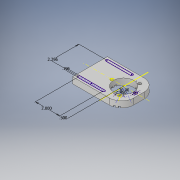
# Autodesk Inventor part: tri_mount
Saved by Autodesk Inventor 2017 (Build 210142000, 142)
## iProperties
Created: 2017-03-10
Part Number: tri_mount
Material: Generic
Document SubType Name: Modeling
Designer: richp
Density: 1 g/cm^3
Appearance: Default
mount_radius: 0.964 in
fov_diameter: 0.300 in
tri_angle: 120.00 deg
hole_diameter: 1.639 in
main_aperture_diameter: 1.639 in
Author: richp
Autodesk Inventor part; units mm, degrees
ref_plane "YZ Plane" through (0, 0, 0) normal (1, 0, 0) x (0, 1, 0)
ref_plane "XZ Plane" through (0, 0, 0) normal (0, 1, 0) x (-1, 0, 0)
ref_plane "XY Plane" through (0, 0, 0) normal (0, 0, 1) x (1, 0, 0)
sketch "Sketch1" plane through (0, 0, 0) normal (0, 1, 0) x (-1, 0, 0)
  line L0 (-54.2742, 0) -> (84.3226, 0) construction
  line L1 (-6.35, -36.068) -> (69.85, -36.068)
  line L2 (69.85, -36.068) -> (69.85, 36.068)
  line L3 (69.85, 36.068) -> (-6.35, 36.068)
  line L4 (-31.75, 10.668) -> (-31.75, -10.668)
  circle A0 centre (0, 0) radius 17 construction
  circle A1 centre (0, 0) radius 20.81
  line L5 (0, 0) -> (-18.9066, 32.7472) construction
  circle A2 centre (0, 0) radius 3.81 construction
  arc A3 (-6.35, 36.068) -> (-31.75, 10.668) centre (-6.35, 10.668) ccw
  arc A4 (-31.75, -10.668) -> (-6.35, -36.068) centre (-6.35, -10.668) ccw
  circle A5 centre (-12.2465, 21.2116) radius 1.6256
  line L6 (0, 0) -> (31.1733, 53.9938) construction
  circle A6 centre (24.493, 0) radius 1.6256
  circle A7 centre (-12.2465, -21.2116) radius 1.6256
  circle A8 centre (-12.2465, 21.2116) radius 3.175 construction
  line L7 (-57.1489, 10.668) -> (-67.0521, 10.668)
  line L8 (-67.0521, 10.668) -> (-67.0521, -7.3902)
  line L9 (-67.0521, -7.3902) -> (-57.1489, -7.3902)
  line L10 (-57.1489, -7.3902) -> (-57.1489, 10.668)
  point P0 (-31.75, -36.068)
  point P1 (-31.75, 36.068)
  dimension "d0" = 72.136
  dimension "d1" = 101.6
  dimension "d2" = 34
  dimension "d3" = 3.81
  dimension "d4" = 31.75
  dimension "tri_angle" = 120
  dimension "fov_diameter" = 7.62
  dimension "d9" = 25.4
  dimension "d12" = 3.2512
  dimension "mount_radius" = 24.493
  dimension "d14" = 60
  dimension "d25" = 6.35
  dimension "main_aperture_diameter" = 41.62
  dimension "d67" = 2.0574
  dimension "d68" = 10.94
  constraints: 22 end point, 9 centre point, 6 point on line, 5 point on circle, 4 coincident, 4 parallel, 4 tangent, 3 horizontal, 2 perpendicular, 2 symmetric about line, 1 equal radius, 3 other
  measures "d0" distance of point (-31.75, 36.068) point (-31.75, -36.068)
  measures "d1" distance of L2.end point (-31.75, 36.068)
  measures "d2" diameter of A0
  measures "d3" radial gap between concentric circles of A1 A0
  measures "d4" distance from line of L5.start L4
  measures "tri_angle" angle of L0 L5
  measures "fov_diameter" diameter of A2
  measures "d9" radius of A3
  measures "d12" diameter of A5
  measures "mount_radius" distance of L5.start A5.centre
  measures "d14" angle of L0 L6
  measures "d25" diameter of A8
  measures "main_aperture_diameter" diameter of A1
  measures "d68" distance edge to line of A1 L4
extrude "Extrusion2" add sketch "Sketch1" against normal blind 12.7 contours A4 L4 A3 L3 L2 L1
sketch "Sketch2" plane through (0, -12.7, 0) normal (0, -1, 0) x (1, 0, 0)
  line L0 (0, 0) -> (-53.7265, 0) construction
  circle A0 centre (0, 0) radius 20.81 projected
  circle A1 centre (12.2465, -21.2116) radius 1.6256 projected
  circle A2 centre (-24.493, 0) radius 1.6256 projected
  circle A3 centre (12.2465, 21.2116) radius 1.6256 projected
  line L1 (-69.85, 36.068) -> (-69.85, -36.068) projected
  line L2 (6.35, 36.068) -> (-69.85, 36.068) projected
  arc A4 (31.75, 10.668) -> (6.35, 36.068) centre (6.35, 10.668) ccw projected
  line L3 (31.75, -10.668) -> (31.75, 10.668) projected
  arc A5 (6.35, -36.068) -> (31.75, -10.668) centre (6.35, -10.668) ccw projected
  line L4 (-69.85, -36.068) -> (6.35, -36.068) projected
  line L5 (54.2742, 0) -> (-84.3226, 0) construction
  line L6 (0, 0) -> (-31.1733, 53.9938) construction
  circle A6 centre (0, 0) radius 17 construction
  circle A7 centre (0, 0) radius 3.81 construction
  line L7 (0, 0) -> (18.9066, 32.7472) construction
  line L8 (41.6502, 64.7743) -> (11.4877, 12.5313) construction
  line L9 (11.4877, 12.5313) -> (41.6502, 64.7743) construction
  line L10 (10.1129, 13.325) -> (40.2754, 65.568)
  line L11 (43.025, 63.9805) -> (12.8625, 11.7375)
  arc A8 (10.1129, 13.325) -> (12.8625, 11.7375) centre (11.4877, 12.5313) ccw
  arc A9 (43.025, 63.9805) -> (40.2754, 65.568) centre (41.6502, 64.7743) ccw
  line L12 (6.4834, 15.4205) -> (36.6459, 67.6635)
  line L13 (33.8962, 69.251) -> (3.7337, 17.008)
  arc A10 (3.7337, 17.008) -> (6.4834, 15.4205) centre (5.1086, 16.2143) ccw
  arc A11 (36.6459, 67.6635) -> (33.8962, 69.251) centre (35.2711, 68.4573) ccw
  line L14 (10.1129, -13.325) -> (40.2754, -65.568)
  line L15 (43.025, -63.9805) -> (12.8625, -11.7375)
  arc A12 (12.8625, -11.7375) -> (10.1129, -13.325) centre (11.4877, -12.5313) ccw
  arc A13 (40.2754, -65.568) -> (43.025, -63.9805) centre (41.6502, -64.7743) ccw
  arc A14 (33.8962, -69.251) -> (36.6459, -67.6635) centre (35.2711, -68.4573) ccw
  line L16 (33.8962, -69.251) -> (3.7337, -17.008)
  arc A15 (6.4834, -15.4205) -> (3.7337, -17.008) centre (5.1086, -16.2143) ccw
  line L17 (6.4834, -15.4205) -> (36.6459, -67.6635)
  line L18 (-16.5962, -2.0955) -> (-76.9212, -2.0955)
  line L19 (-76.9212, -5.2705) -> (-16.5962, -5.2705)
  arc A16 (-16.5962, -5.2705) -> (-16.5962, -2.0955) centre (-16.5962, -3.683) ccw
  arc A17 (-76.9212, -2.0955) -> (-76.9212, -5.2705) centre (-76.9212, -3.683) ccw
  arc A18 (-76.9212, 5.2705) -> (-76.9212, 2.0955) centre (-76.9212, 3.683) ccw
  line L20 (-76.9212, 5.2705) -> (-16.5962, 5.2705)
  arc A19 (-16.5962, 2.0955) -> (-16.5962, 5.2705) centre (-16.5962, 3.683) ccw
  line L21 (-16.5962, 2.0955) -> (-76.9212, 2.0955)
  point P0 (26.5689, 38.6528)
  dimension "d20" = 3.683
  dimension "pin_diameter" = 3.175
  dimension "d28" = 63.5
  constraints: 32 end point, 27 symmetric about line, 24 point on circle, 12 centre point, 4 tangent, 2 parallel, 1 collinear, 1 horizontal, 1 midpoint, 12 other
  measures "d20" distance between parallel lines of L8 L7
  measures "pin_diameter" distance between parallel lines of L10 L11
extrude "Extrusion3" cut sketch "Sketch2" against normal blind 2.921 contours L11 A8 L10 A0 | A0 L10 A4 L11 | L15 A5 L14 A0 | A0 L14 A12 L15 | A4 L10 A9 L11 | L15 A13 L14 A5 | L12 A10 L13 A0 | A0 L13 A4 L12 | L17 A5 L16 A0 | A0 L16 A15 L17 | A4 L13 A11 L12 | L17 A14 L16 A5 | L20 A19 L21 A0 | A0 L21 L1 L20 | L19 L1 L18 A0 | A0 L18 A16 L19 | L1 L21 A18 L20 | L19 A17 L18 L1
sketch "Sketch3" plane through (0, 0, 0) normal (0, 1, 0) x (1, 0, 0)
  circle A0 centre (12.2465, -21.2116) radius 3.175 construction
  circle A1 centre (12.2465, -21.2116) radius 3.175
  line L0 (54.2742, 0) -> (-84.3226, 0) construction
  line L1 (0, 0) -> (-31.1733, -53.9938) construction
  circle A2 centre (12.2465, 21.2116) radius 3.175
  circle A3 centre (-24.493, 0) radius 3.175
  constraints: 3 centre point, 2 symmetric about line, 1 coincident, 1 concentric, 2 other
extrude "Extrusion4" cut sketch "Sketch3" against normal blind 9.779
sketch "Sketch4" plane through (0, 0, 0) normal (0, 1, 0) x (1, 0, 0)
  line L0 (54.2742, 0) -> (-84.3226, 0) construction
  line L1 (-63.5, -29.1592) -> (-12.7, -29.1592) construction
  line L2 (-63.5, -26.67) -> (-12.7, -26.67)
  line L3 (-12.7, -31.6484) -> (-63.5, -31.6484)
  arc A0 (-63.5, -26.67) -> (-63.5, -31.6484) centre (-63.5, -29.1592) ccw
  arc A1 (-12.7, -31.6484) -> (-12.7, -26.67) centre (-12.7, -29.1592) ccw
  line L4 (-63.5, 26.67) -> (-12.7, 26.67)
  line L5 (-12.7, 31.6484) -> (-63.5, 31.6484)
  arc A2 (-63.5, 31.6484) -> (-63.5, 26.67) centre (-63.5, 29.1592) ccw
  arc A3 (-12.7, 26.67) -> (-12.7, 31.6484) centre (-12.7, 29.1592) ccw
  point P0 (0, 0)
  point P1 (-38.1, -29.1592)
  dimension "d33" = 4.9784
  dimension "d34" = 50.8
  dimension "d35" = 58.3184
  dimension "d36" = 12.7
  constraints: 12 end point, 8 point on circle, 6 symmetric about line, 4 centre point, 4 tangent, 1 horizontal, 1 midpoint, 1 parallel, 2 other
  measures "d33" distance between parallel lines of L2 L3
  measures "d34" distance of L1.end L1.start
  measures "d35" distance from line of L1 A2.centre
  measures "d36" horizontal distance of L1.end point (0, 0)
sketch "Sketch5" plane through (0, -12.7, 0) normal (0, -1, 0) x (1, 0, 0)
  circle A0 centre (12.2465, 21.2116) radius 1.6256 projected
  line L0 (0, 0) -> (18.9066, 32.7472) construction
  line L1 (54.2742, 0) -> (-84.3226, 0) construction
  line L2 (0, 0) -> (-31.1733, 53.9938) construction
  circle A1 centre (12.2465, 21.2116) radius 3.175 construction
  line L3 (9.4969, 22.7991) -> (6.9569, 18.3997)
  line L4 (14.9961, 19.6241) -> (12.4561, 15.2247)
  line L5 (6.9569, 18.3997) -> (12.4561, 15.2247)
  arc A2 (14.9961, 19.6241) -> (9.4969, 22.7991) centre (12.2465, 21.2116) ccw
  line L6 (-24.493, 3.175) -> (-19.413, 3.175)
  line L7 (-24.493, -3.175) -> (-19.413, -3.175)
  line L8 (-19.413, 3.175) -> (-19.413, -3.175)
  arc A3 (-24.493, 3.175) -> (-24.493, -3.175) centre (-24.493, 0) ccw
  line L9 (9.4969, -22.7991) -> (6.9569, -18.3997)
  line L10 (14.9961, -19.6241) -> (12.4561, -15.2247)
  line L11 (6.9569, -18.3997) -> (12.4561, -15.2247)
  arc A4 (9.4969, -22.7991) -> (14.9961, -19.6241) centre (12.2465, -21.2116) ccw
  dimension "d50" = 5.08
  constraints: 18 end point, 10 symmetric about line, 8 point on circle, 4 tangent, 3 centre point, 2 parallel, 1 perpendicular, 2 other
  measures "d50" distance from line of A0.centre L5
extrude "Extrusion6" [suppressed]
extrude "Extrusion7" [suppressed]
sketch "Sketch6" plane through (0, 0, 0) normal (0, 1, 0) x (1, 0, 0)
  line L0 (0, 0) -> (18.9066, -32.7472) construction
  line L1 (41.6502, -64.7743) -> (11.4877, -12.5313) construction
  line L2 (0, 0) -> (33.579, -42.2146) construction
  circle A0 centre (15.5113, -19.5004) radius 3.175
  circle A1 centre (9.1322, -23.1834) radius 3.175
  line L3 (0, 0) -> (-31.1733, -53.9938) construction
  line L4 (54.2742, 0) -> (-84.3226, 0) construction
  circle A2 centre (-24.6435, 3.683) radius 3.175
  circle A3 centre (-24.6435, -3.683) radius 3.175
  circle A4 centre (15.5113, 19.5004) radius 3.175
  circle A5 centre (9.1322, 23.1834) radius 3.175
  dimension "d45" = 8.5
  dimension "d46" = 6.35
  constraints: 6 centre point, 5 symmetric about line, 2 end point, 2 point on line, 5 other
  measures "d45" angle of L2 L0
  measures "d46" diameter of A0
extrude "Extrusion8" [suppressed]
chamfer "Chamfer2" [suppressed]
sketch "Sketch7" plane through (0, -12.7, 0) normal (0, -1, 0) x (1, 0, 0)
  line L0 (0, 0) -> (-31.1733, 53.9938) construction
  line L1 (0, 0) -> (18.9066, 32.7472) construction
  circle A0 centre (12.2465, 21.2116) radius 3.175
  circle A1 centre (-24.493, 0) radius 3.175
  line L2 (54.2742, 0) -> (-84.3226, 0) construction
  circle A2 centre (12.2465, -21.2116) radius 3.175
  dimension "d54" = 6.35
  constraints: 3 centre point, 2 symmetric about line, 1 coincident, 2 other
  measures "d54" diameter of A0
extrude "Extrusion9" cut sketch "Sketch7" against normal blind 2.159
sketch "Sketch8" plane through (0, 0, 0) normal (0, 1, 0) x (1, 0, 0)
  circle A0 centre (0, 0) radius 20.81 projected
  line L0 (54.2742, 0) -> (-84.3226, 0) construction
  line L1 (0, 0) -> (12.8396, -66.0541) construction
  point P0 (4.3134, -22.1907)
  point P1 (4.3134, 22.1907)
  dimension "d57" = 101
  dimension "d58" = 22.606
  constraints: 2 end point, 1 point on line, 1 symmetric about line
  measures "d57" angle of L1 L0
  measures "d58" distance of point (0, 0) point (4.313, -22.191)
hole "Hole1" at (4.3134, 0, 22.1907) at (4.3134, 0, -22.1907) direction (0, -1, 0) diameter 1.27 depth 25.4 tip angle 118
sketch "Sketch9" plane through (0, 0, 0) normal (0, 1, 0) x (1, 0, 0)
  line L0 (0, 0) -> (22.9874, -39.8154) construction
  line L1 (15.2539, -22.2295) -> (20.6849, -31.6363) projected
  circle A0 centre (12.2465, -21.2116) radius 3.175 projected
  line L2 (12.2465, -21.2116) -> (22.1452, -15.4966) construction
  point P0 (17.1958, -18.3541)
  point P1 (7.2972, -24.0691)
  dimension "d69" = 11.43
  constraints: 4 end point, 1 midpoint, 1 parallel, 1 perpendicular, 1 symmetric about line, 1 other
  measures "d69" distance of point (17.196, -18.354) point (7.297, -24.069)
hole "Hole2" at (17.1958, 0, 18.3541) at (7.2972, 0, 24.0691) direction (0, -1, 0) diameter 1.7018 depth 12.7 tip angle 118
sketch "Sketch10" plane through (0, 0, 0) normal (0, 1, 0) x (1, 0, 0)
  circle A0 centre (-24.493, 0) radius 3.175 projected
  line L0 (0, 50.4952) -> (0, -50.4952) projected
  line L1 (0, 0) -> (18.9066, -32.7472) construction
  circle A1 centre (24.493, 0) radius 3.175
  line L2 (0, 0) -> (37.8406, -21.8473) construction
  point P0 (7.2972, -24.0691)
  point P1 (17.1958, -18.3541)
  point P2 (24.493, 5.715)
  point P3 (24.493, -5.715)
  dimension "d77" = 30
  constraints: 3 symmetric about line, 2 end point, 1 centre point, 1 other
  measures "d77" angle of L2 L1
extrude "Extrusion10" cut sketch "Sketch10" against normal blind 25.4 contours A1
sketch "Sketch11" plane through (0, 0, 0) normal (0, 1, 0) x (1, 0, 0)
  point P0 (0, 0)
  point P1 (24.493, -5.715)
  point P2 (24.493, 5.715)
hole "Hole3" at (24.493, 0, 5.715) at (24.493, 0, -5.715) direction (0, -1, 0) diameter 1.7018 depth 12.7 tip angle 118
equation "\"fov_diameter\" = 2 * d3"
equation "\"d14\" = 0.5 * tri_angle"
equation "\"d15\" = plate_thickness"
equation "\"d23\" = pin_depth"
equation "\"d26\" = magnet_depth"
equation "\"d40\" = bearing_relief_depth"
equation "\"d46\" = magnet_diameter"
equation "\"d47\" = magnet_depth"
equation "\"d54\" = magnet_diameter"
equation "\"d55\" = bearing_relief_depth"
equation "\"plate_thickness\" = 12.7"
equation "\"magnet_depth\" = plate_thickness - pin_depth"
equation "\"hole_diameter\" = d2 + fov_diameter"
equation "\"pin_depth\" = 2.921"
equation "\"bearing_relief_depth\" = 2.159"
equation "\"magnet_diameter\" = 6.35"
body "Solid2"
